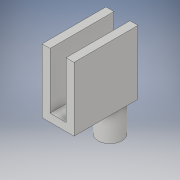
# Autodesk Inventor part: coffee
Saved by Autodesk Inventor 2017 (Build 210142000, 142)
## iProperties
Created: 2019-12-05
Part Number: coffee
Material: Generic
Document SubType Name: Modeling
Designer: Christian
Density: 1 g/cm^3
Appearance: Default
Author: Christian
Autodesk Inventor part; units mm, degrees
ref_plane "YZ Plane" through (0, 0, 0) normal (1, 0, 0) x (0, 1, 0)
ref_plane "XZ Plane" through (0, 0, 0) normal (0, 1, 0) x (-1, 0, 0)
ref_plane "XY Plane" through (0, 0, 0) normal (0, 0, 1) x (1, 0, 0)
sketch "Body_Skt" plane through (0, 0, 0) normal (0, 0, 1) x (1, 0, 0)
  line L0 (-2, -4) -> (2, -4)
  line L1 (2, -4) -> (2, 4)
  line L2 (2, 4) -> (-2, 4)
  line L3 (-2, 4) -> (-2, -4)
  line L4 (-2, -4) -> (2, 4) construction
  line L5 (2, -4) -> (-2, 4) construction
  point P0 (0, 0)
  dimension "d0" = 4
  dimension "d1" = 8
  constraints: 12 end point, 2 midpoint, 2 parallel, 1 horizontal, 1 perpendicular
  measures "d0" distance of L1.end L2.end
  measures "d1" distance of L0.end L1.end
extrude "Body" add sketch "Body_Skt" along normal blind 8
sketch "Wall_Skt" plane through (-2, -4, 0) normal (0, -1, 0) x (1, 0, 0)
  line L0 (0, 8) -> (4, 8) projected
  line L1 (3, 8) -> (1, 8)
  line L2 (1, 8) -> (1, 1)
  line L3 (1, 1) -> (3, 1)
  line L4 (3, 1) -> (3, 8)
  line L5 (4, 0) -> (4, 8) projected
  line L6 (0, 0) -> (4, 0) projected
  line L7 (0, 0) -> (0, 8) projected
  point P0 (2, 0)
  dimension "d4" = 1
  dimension "d5" = 1
  dimension "d6" = 1
  constraints: 8 end point, 2 parallel, 1 horizontal, 1 perpendicular, 1 point on line
  measures "d4" distance between parallel lines of L5 L4
  measures "d5" distance between parallel lines of L6 L3
  measures "d6" distance between parallel lines of L7 L2
extrude "Wall" cut sketch "Wall_Skt" against normal through all contours L0 L4 L3 L2
sketch "Leg_Skt" plane through (0, 0, 0) normal (0, 0, -1) x (-1, 0, 0)
  circle A0 centre (0, 2.5) radius 1.5
  line L0 (-2, 4) -> (2, 4) projected
  line L1 (0, 0) -> (0, 4) construction
  dimension "d10" = 3
  constraints: 2 end point, 1 centre point, 1 midpoint, 1 point on line, 1 tangent
  measures "d10" diameter of A0
extrude "Leg" add sketch "Leg_Skt" along normal blind 4
equation "\"d0\" = wall_inner_diam + 2 * wall_outer_diam"
equation "\"d1\" = wall_widh"
equation "\"d2\" = wall_height"
equation "\"d4\" = wall_outer_diam"
equation "\"d5\" = wall_outer_diam"
equation "\"d6\" = wall_outer_diam"
equation "\"d7\" = d1 - wall_outer_diam"
equation "\"d10\" = leg_diam"
equation "\"d11\" = leg_height"
equation "\"wall_inner_diam\" = 2"
equation "\"wall_outer_diam\" = 1"
equation "\"wall_height\" = 8"
equation "\"leg_diam\" = 3"
equation "\"leg_height\" = 4"
equation "\"wall_widh\" = 8"
body "Solid1"
